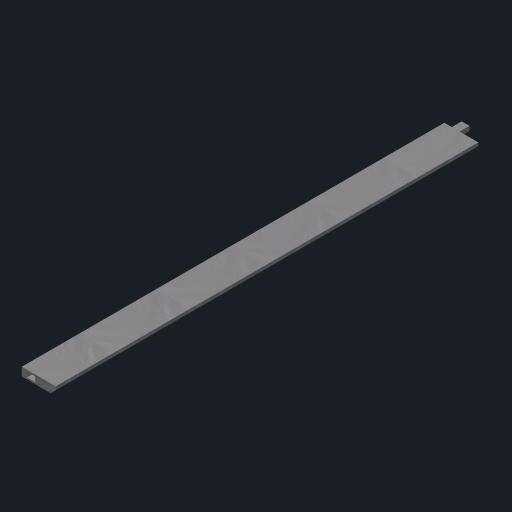
# Autodesk Inventor part: SEPARADOR
Saved by Autodesk Inventor 2024.3 (Build 283343000, 343)
## iProperties
Created: 2024-07-03
Part Number: SEPARADOR
Material: Steel, Mild, Welded
Document SubType Name: Modeling
Designer: Niler
Density: 7.85 g/cm^3
Appearance: Weld - Steel Mild
Author: Niler
Autodesk Inventor part; units mm, degrees
ref_plane "YZ Plane" through (0, 0, 0) normal (1, 0, 0) x (0, 1, 0)
ref_plane "XZ Plane" through (0, 0, 0) normal (0, 1, 0) x (-1, 0, 0)
ref_plane "XY Plane" through (0, 0, 0) normal (0, 0, 1) x (1, 0, 0)
sketch "Sketch1" plane through (0, 0, 0) normal (0, 1, 0) x (-1, 0, 0)
  line L0 (-10, 124.5) -> (10, 124.5)
  line L1 (10, 124.5) -> (10, -124.5)
  line L2 (10, -124.5) -> (-10, -124.5)
  line L3 (-10, -124.5) -> (-10, 124.5)
  line L4 (-10, 124.5) -> (10, -124.5) construction
  line L5 (10, 124.5) -> (-10, -124.5) construction
  point P0 (0, 0)
  dimension "d0" = 20
  dimension "d1" = 249
  constraints: 12 end point, 2 midpoint, 2 parallel, 1 horizontal, 1 perpendicular
  measures "d0" distance of L1.end L2.end
  measures "d1" distance of L0.end L1.end
extrude "Extrusion1" add sketch "Sketch1" along normal blind 5
chamfer "Chamfer1" distance 3 angle 45 1 edges at (10, 0, 0)
sketch "Sketch3" plane through (-10, 5, 124.5) normal (0, 0, 1) x (1, 0, 0)
  line L0 (20, -2) -> (17, -5) projected
  line L1 (20, -2) -> (20, 0) projected
  line L2 (0, 0) -> (20, 0) projected
  line L3 (0, -5) -> (0, 0) projected
  line L4 (0, -5) -> (17, -5) projected
  line L5 (3, -4) -> (8, -4)
  line L6 (8, -4) -> (8, -1)
  line L7 (8, -1) -> (3, -1)
  line L8 (3, -1) -> (3, -4)
  line L9 (3, -4) -> (8, -1) construction
  line L10 (8, -4) -> (3, -1) construction
  point P0 (10, -5)
  point P1 (5.5, -2.5)
  point P2 (0, -2.5)
  dimension "d10" = 5
  dimension "d11" = 3
  dimension "d12" = 3
  constraints: 12 end point, 3 midpoint, 2 parallel, 1 horizontal, 1 horizontal alignment, 1 perpendicular
  measures "d10" distance of L7.end L6.end
  measures "d11" distance of L6.end L5.end
  measures "d12" distance between parallel lines of L3 L8
extrude "Extrusion3" cut sketch "Sketch3" against normal blind 7.1 contours L8 L7 L6 L5
sketch "Sketch4" plane through (10, 5, -124.5) normal (0, 0, -1) x (-1, 0, 0)
  line L0 (12, -1) -> (12, -4) projected
  line L1 (17, -1) -> (12, -1) projected
  line L2 (17, -4) -> (17, -1) projected
  line L3 (12, -4) -> (17, -4) projected
  line L4 (12.2, -1.2) -> (12.2, -3.8)
  line L5 (12.2, -3.8) -> (16.8, -3.8)
  line L6 (16.8, -3.8) -> (16.8, -1.2)
  line L7 (16.8, -1.2) -> (12.2, -1.2)
  point P0 (10, -5)
  dimension "d15" = 0.2
  constraints: 8 end point, 3 other
  measures "d15" distance between parallel lines of L1 L7
extrude "Extrusion4" add sketch "Sketch4" along normal blind 7 contours L7 L6 L5 L4
body "Solid1"
